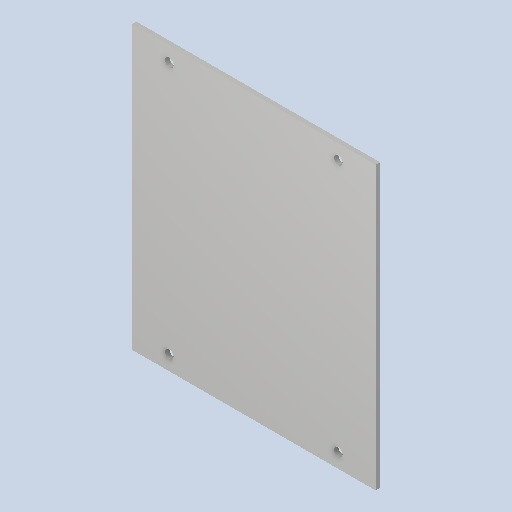
# Autodesk Inventor part: memesat shear panel type 2
Saved by Autodesk Inventor 2022 (Build 260153000, 153)
## iProperties
Created: 2020-02-20
Part Number: memesat shear panel type 2
Material: Aluminum 6061
Document SubType Name: Modeling
Designer: UGA SSRL
Density: 2.7 g/cm^3
Appearance: Aluminum - Flat
Mass: 25.6903 g
Surface Area: 110.966 cm^2
Volume: 9.51491 cm^3
Author: UGA SSRL
Autodesk Inventor part; units mm, degrees
ref_plane "YZ Plane" through (0, 0, 0) normal (1, 0, 0) x (0, 1, 0)
ref_plane "XZ Plane" through (0, 0, 0) normal (0, 1, 0) x (-1, 0, 0)
ref_plane "XY Plane" through (0, 0, 0) normal (0, 0, 1) x (1, 0, 0)
sketch "Sketch1" plane through (0, 0, 0) normal (0, 0, 1) x (1, 0, 0)
  line L0 (-41.5, 48) -> (41.5, 48)
  line L1 (41.5, 48) -> (41.5, -48)
  line L2 (41.5, -48) -> (-41.5, -48)
  line L3 (-41.5, -48) -> (-41.5, 48)
  point P0 (0, 0)
  dimension "d0" = 83
  dimension "d1" = 96
  dimension "d2" = 48
  dimension "d3" = 41.5
  constraints: 8 end point, 2 parallel, 1 horizontal, 1 perpendicular
  measures "d0" distance of L1.end L2.end
  measures "d1" distance of L0.end L1.end
  measures "d2" distance from line of L0 point (0, 0)
  measures "d3" distance from line of point (0, 0) L3
extrude "Extrusion1" add sketch "Sketch1" against normal blind 1.5
sketch "Sketch2" plane through (0, 0, 0) normal (0, 0, 1) x (1, 0, 0)
  line L0 (-41.5, 48) -> (41.5, 48) projected
  line L1 (0, 0) -> (16.5924, 0) construction
  point P0 (-28.75, 43)
  point P1 (28.75, 43)
  point P2 (-28.75, -43)
  point P3 (28.75, -43)
  dimension "d6" = 57.5
  dimension "d7" = 5
  dimension "d21" = 28.75
  constraints: 2 end point, 2 symmetric about line, 1 horizontal, 1 horizontal alignment
  measures "d6" distance of point (-28.75, 43) point (28.75, 43)
  measures "d7" distance from line of L0 point (-28.75, 43)
  measures "d21" horizontal distance of L1.start point (-28.75, 43)
hole "Hole1" at (-28.75, 43, 0) at (28.75, 43, 0) at (-28.75, -43, 0) at (28.75, -43, 0) direction (0, 0, -1) diameter 2.946 end through all clearance for "Flat Head Machine Screw (100)" size "#4" standard "Ansi Unified Screw Threads"
equation "\"d2\" = 0.5 * d1"
equation "\"d3\" = 0.5 * d0"
equation "\"d21\" = 0.5 * d6"
body "Solid1"
